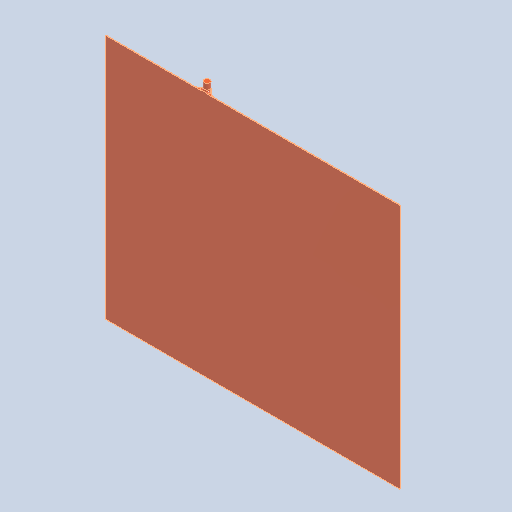
# Autodesk Inventor part: Bed Heater
Saved by Autodesk Inventor 2024 (Build 280153000, 153)
## iProperties
Created: 2024-08-02
Part Number: Bed Heater
Material: Rubber
Document SubType Name: Modeling
Designer: Ishaan
Density: 0.93 g/cm^3
Appearance: Smooth - Light Orange
Author: Ishaan
Autodesk Inventor part; units mm, degrees
ref_plane "YZ Plane" through (0, 0, 0) normal (1, 0, 0) x (0, 1, 0)
ref_plane "XZ Plane" through (0, 0, 0) normal (0, 1, 0) x (-1, 0, 0)
ref_plane "XY Plane" through (0, 0, 0) normal (0, 0, 1) x (1, 0, 0)
sketch "Sketch1" plane through (0, 0, 0) normal (0, 0, 1) x (1, 0, 0)
  line L0 (150, -125) -> (-150, -125)
  line L1 (-150, -125) -> (-150, 125)
  line L2 (-150, 125) -> (150, 125)
  line L3 (150, 125) -> (150, -125)
  line L4 (150, -125) -> (-150, 125) construction
  line L5 (-150, -125) -> (150, 125) construction
  point P0 (0, 0)
  dimension "d0" = 300
  dimension "d1" = 250
  constraints: 12 end point, 2 midpoint, 2 parallel, 1 horizontal, 1 perpendicular
  measures "d0" distance of L1.end L2.end
  measures "d1" distance of L0.end L1.end
extrude "Extrusion1" add sketch "Sketch1" along normal blind 1
fillet "Fillet1" radius 1 4 edges at (150, -125, 0.5) (-150, -125, 0.5) (-150, 125, 0.5) (150, 125, 0.5)
sketch "Sketch2" plane through (-149, 125, 0) normal (0, 1, 0) x (1, 0, 0)
  circle A0 centre (99, 2.5) radius 3
  line L0 (298, -1) -> (0, -1) projected
  line L1 (298, 0) -> (0, 0) projected
  point P0 (149, 0)
  point P1 (149, 0)
  point P2 (97.3417, 0)
  point P3 (100.6583, 0)
  dimension "d6" = 6
  dimension "d7" = 3.5
  dimension "d8" = 50
  constraints: 1 centre point, 1 midpoint
  measures "d6" diameter of A0
  measures "d7" distance from line of L0 A0.centre
  measures "d8" horizontal distance of point (149, 0) A0.centre
extrude "Extrusion2" add sketch "Sketch2" along normal blind 8 and the other way blind 30
fillet "Fillet3" radius 3 1 edges at (-50, 95, -5.5)
fillet "Fillet4" radius 10 4 edges at (-48.3417, 111.5, 0) (-51.6583, 111.5, 0) (-48.8246, 96.8302, 0) (-51.1754, 96.8302, 0)
fillet "Fillet5" radius 2 2 edges at (-52.9488, 125, -1.9479) (-47.8479, 125, -0.41)
fillet "Fillet6" radius 0.5 13 edges at (-42.3521, 125, -0.4514) (-46.586, 125.7234, -3.0648) (149.7071, 124.7071, 0) (150, 0, 0) (149.7071, -124.7071, 0) (0, -125, 0) (-149.7071, -124.7071, 0) (-150, 0, 0) (-149.7071, 124.7071, 0) (-104.8092, 125, 0) (-57.6479, 125, -0.4514) (-53.414, 125.7234, -3.0648) (54.8092, 125, 0)
body "Solid1"
